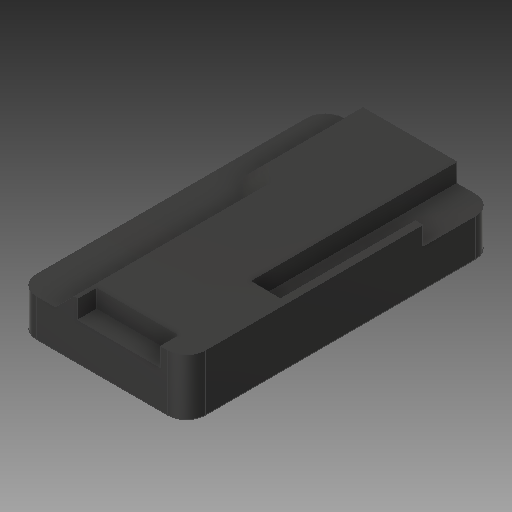
# Autodesk Inventor part: APM
Saved by Autodesk Inventor 2019 (Build 230136000, 136)
## iProperties
Created: 2020-03-12
Part Number: APM
Material: ABS Plastic
Document SubType Name: Modeling
Designer: Pulag
Density: 1.06 g/cm^3
Appearance: Smooth - White
Author: Pulag
Autodesk Inventor part; units mm, degrees
ref_plane "YZ Plane" through (0, 0, 0) normal (1, 0, 0) x (0, 1, 0)
ref_plane "XZ Plane" through (0, 0, 0) normal (0, 1, 0) x (-1, 0, 0)
ref_plane "XY Plane" through (0, 0, 0) normal (0, 0, 1) x (1, 0, 0)
sketch "Sketch1" plane through (0, 0, 0) normal (0, 1, 0) x (-1, 0, 0)
  line L0 (-22.5, 41) -> (22.5, 41)
  line L1 (22.5, 41) -> (22.5, -41)
  line L2 (22.5, -41) -> (-22.5, -41)
  line L3 (-22.5, -41) -> (-22.5, 41)
  line L4 (-22.5, 41) -> (22.5, -41) construction
  line L5 (22.5, 41) -> (-22.5, -41) construction
  point P0 (0, 0)
  dimension "d0" = 45
  dimension "d1" = 82
  constraints: 12 end point, 2 midpoint, 2 parallel, 1 horizontal, 1 perpendicular
  measures "d0" distance of L1.end L2.end
  measures "d1" distance of L0.end L1.end
extrude "Extrusion1" add sketch "Sketch1" along normal blind 10
sketch "Sketch2" plane through (0, 10, 0) normal (0, 1, 0) x (1, 0, 0)
  line L0 (22.5, -41) -> (22.5, 41) projected
  line L1 (22.5, 41) -> (-22.5, 41) projected
  line L2 (12.5, 41) -> (12.5, -14)
  line L3 (12.5, -14) -> (20.5, -14)
  line L4 (20.5, -14) -> (20.5, 22)
  line L5 (20.5, 22) -> (22.5, 22)
  line L6 (-22.5, -41) -> (22.5, -41) projected
  line L7 (22.5, -41) -> (22.5, 22)
  line L8 (22.5, -41) -> (15.5, -41)
  line L9 (15.5, -41) -> (15.5, -36)
  line L10 (-22.5, -41) -> (-12.5, -41)
  line L11 (-12.5, -41) -> (-12.5, -36)
  line L12 (-12.5, -36) -> (-12.5, 9)
  line L13 (-17.5, 41) -> (12.5, 41)
  line L14 (15.5, -36) -> (-6.5, -36)
  line L15 (-6.5, -36) -> (-6.5, -41)
  line L16 (-12.5, -41) -> (-6.5, -41)
  line L17 (-12.5, 9) -> (-17.5, 14)
  line L18 (-12.5, 9) -> (-5.4289, 9) construction
  line L19 (-17.5, 14) -> (-17.5, 41)
  point P0 (0, 0)
  dimension "d6" = 10
  dimension "d7" = 55
  dimension "d8" = 8
  dimension "d9" = 36
  dimension "d10" = 90
  dimension "d11" = 7
  dimension "d12" = 5
  dimension "d13" = 90
  dimension "d14" = 28
  dimension "d15" = 10
  dimension "d21" = 22
  dimension "d29" = 135
  constraints: 34 end point, 7 perpendicular, 6 point on line, 3 vertical, 2 horizontal, 1 equal length
  measures "d6" distance of L0.end L2.start
  measures "d7" distance of L2.start L2.end
  measures "d8" distance of L2.end L3.end
  measures "d9" distance of L3.end L4.end
  measures "d10" angle of L4 L3
  measures "d11" distance of L0.start L8.end
  measures "d12" distance of L8.end L9.end
  measures "d13" angle of L8 L9
  measures "d14" distance of L9.end L11.end
  measures "d15" distance of L6.start L10.end
  measures "d21" distance of L9.end L14.end
  measures "d29" angle of L18 L17
extrude "Extrusion2" add sketch "Sketch2" along normal blind 5 contours L6 L9 L14 L15 L11 L12 L17 L19 L1 L2 L3 L4 L5 L0
fillet "Fillet3" radius 5 4 edges at (22.5, 7.5, 41) (-22.5, 5, 41) (22.5, 5, -41) (-22.5, 5, -41)
draft "FaceDraft3" angle 45 pull direction (0, 1, 0) faces at (-15.8333, 11.6667, -12.3333) fixed edges at (-15, 10, -11.5)
draft "FaceDraft4" angle 45 pull direction (0, 1, 0) faces at (-17.5, 11.6667, -25.357) fixed edges at (-17.5, 10, -27.5)
draft "FaceDraft5" angle 45 pull direction (0, 1, 0) faces at (-12.5, 13.3333, 5.3096) fixed edges at (-12.5, 10, 16)
body "Solid1"
